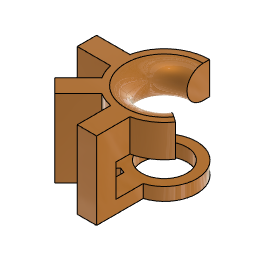
Exercise-18 v0 (Autodesk Fusion 360 design; units mm, degrees)
Autodesk Fusion 360 part; units mm, degrees
sketch "Sketch1" plane through (0, 0, 0) normal (1, 0, 0) x (0, 1, 0)
  line L0 (0, -2.5) -> (1, -2.5)
  line L1 (1, -2.5) -> (1, 2.5)
  line L2 (1, 2.5) -> (0, 2.5)
  arc A0 (0, 2.5) -> (0, -2.5) centre (0, 0) ccw
  line L3 (-6, 5) -> (-6, -5)
  dimension "d1" = 5
  dimension "d2" = 1
  dimension "d3" = 5
  dimension "d4" = 6
  constraint coincident A0.centre origin
  constraint horizontal L0
  constraint vertical L1
  constraint horizontal L2
  constraint vertical L3
  measures "d1" diameter of A0
  measures "d2" distance of L0.start L0.end
  measures "d3" distance of L0.start L2.end
  measures "d4" distance of A0.centre L3
revolve "Revolve1" add sketch "Sketch1" angle 235 about axis through (0, -6, 5) along (0, 0, 1) makes body 1
sketch "Sketch2" plane through (0, 0, 2.5) normal (0, 0, 1) x (-1, 0, 0)
  line L0 (0, 0) -> (0, -1)
  arc A0 (0, -1) -> (-5.7341, 10.015) centre (0, 6) ccw
  line L1 (-5.7341, 10.015) -> (-4.9149, 9.4415)
  arc A1 (0, 0) -> (-4.9149, 9.4415) centre (0, 6) ccw
  line L2 (6, 7.5) -> (12, 7.5)
  line L3 (12, 7.5) -> (12, 4.5)
  line L4 (12, 4.5) -> (6, 4.5)
  line L5 (6, 4.5) -> (6, 7.5)
  line L6 (12, 7.5) -> (9, 7.5)
  line L7 (9, 7.5) -> (9, 4.5)
  line L8 (9, 4.5) -> (12, 4.5)
  line L9 (12, 4.5) -> (12, 7.5)
  line L10 (7.4246, 15.5459) -> (5.3033, 13.4246)
  line L11 (5.3033, 13.4246) -> (7.4246, 11.3033)
  line L12 (9.5459, 13.4246) -> (7.4246, 15.5459)
  line L13 (7.4246, 11.3033) -> (9.5459, 13.4246)
  line L14 (7.4246, 15.5459) -> (9.5459, 13.4246)
  line L15 (5.3033, 9.182) -> (3.182, 11.3033)
  line L16 (3.182, 11.3033) -> (7.4246, 15.5459)
  line L17 (9.5459, 13.4246) -> (5.3033, 9.182)
  line L18 (-1.5, 18) -> (-1.5, 15)
  line L19 (-1.5, 15) -> (1.5, 15)
  line L20 (1.5, 18) -> (-1.5, 18)
  line L21 (1.5, 15) -> (1.5, 18)
  line L22 (-1.5, 18) -> (1.5, 18)
  line L23 (1.5, 12) -> (-1.5, 12)
  line L24 (-1.5, 12) -> (-1.5, 18)
  line L25 (1.5, 18) -> (1.5, 12)
  dimension "d6" = 6
  dimension "d7" = 3
  dimension "d8" = 12
  dimension "d9" = 1.5
  dimension "d10" = 3
  dimension "d11" = 3
  dimension "d13" = 90
  constraint horizontal L2
  constraint vertical L3
  constraint horizontal L4
  constraint vertical L5
  constraint horizontal L6
  constraint vertical L7
  constraint horizontal L8
  constraint vertical L9
  measures "d6" distance of L2.start L2.end
  measures "d7" distance of L2.start L4.end
  measures "d8" distance of A0.centre L3
  measures "d9" distance of A0.centre L4
  measures "d10" distance of L2.end L6.end
  measures "d11" distance of L2.end L3.end
extrude "Extrude1" add sketch "Sketch2" against normal blind 12 separate body contours L2 L3 L4 L6 L7 L8 L9 | L10 L11 L12 L13 L14 L16 L17 | L18 L19 L20 L21 L22 L24 L25 makes body 2 at (-6.0104, -14.1317, -5.5) makes body 3 at (0.5, -15, -1.5) makes body 4 at (-9, -6.5, -1.5)
extrude "Extrude2" add sketch "Sketch2" against normal blind 5 contours A0 L2 L4 L7 | A0 L11 L16 L17 | A0 L19 L24 L25 bodies 1 2 3 4
sketch "Sketch3" plane through (0, 0, -9.5) normal (0, 0, -1) x (1, 0, 0)
  line L0 (-1.5, 15) -> (1.5, 15)
  line L1 (1.5, 15) -> (1.5, 18)
  line L2 (1.5, 18) -> (-1.5, 18)
  line L3 (-1.5, 18) -> (-1.5, 15)
  line L4 (-12, 7.5) -> (-6.8374, 7.5)
  line L5 (-6.8374, 4.5) -> (-12, 4.5)
  line L6 (-12, 4.5) -> (-12, 7.5)
  arc A0 (-6.8374, 4.5) -> (0, -1) centre (0, 6) ccw
  line L7 (-1.5, 18) -> (-1.5, 12.8374)
  line L8 (1.5, 18) -> (-1.5, 18)
  line L9 (1.5, 12.8374) -> (1.5, 18)
  arc A1 (-1.5, 12.8374) -> (-3.7741, 11.8954) centre (0, 6) ccw
  line L10 (-9.5459, 13.4246) -> (-5.8954, 9.7741)
  line L11 (-7.4246, 15.5459) -> (-9.5459, 13.4246)
  line L12 (-3.7741, 11.8954) -> (-7.4246, 15.5459)
  arc A2 (-5.8954, 9.7741) -> (-6.8374, 7.5) centre (0, 6) ccw
  arc A3 (5.7341, 10.015) -> (1.5, 12.8374) centre (0, 6) ccw
  line L13 (0, -1) -> (0, 0)
  line L14 (4.9149, 9.4415) -> (5.7341, 10.015)
  line L15 (0, 0) -> (0, 2.5)
  line L16 (2.867, 8.0075) -> (4.9149, 9.4415)
  arc A4 (2.867, 8.0075) -> (0, 2.5) centre (0, 6) ccw
  circle A5 centre (0, 6) radius 3.5
  circle A6 centre (0, 6) radius 5
  line L17 (1.5, 12.8374) -> (-1.5, 12.8374)
  line L18 (-1.5, 12.8374) -> (-1.5, 9.8374)
  line L19 (-1.5, 9.8374) -> (1.5, 9.8374)
  line L20 (1.5, 9.8374) -> (1.5, 12.8374)
  line L21 (-3.7741, 7.6528) -> (-1.6528, 9.7741)
  line L22 (-1.6528, 9.7741) -> (-3.7741, 11.8954)
  line L23 (-5.8954, 9.7741) -> (-3.7741, 7.6528)
  line L24 (-3.7741, 11.8954) -> (-5.8954, 9.7741)
  line L25 (-3.8374, 4.5) -> (-3.8374, 7.5)
  line L26 (-3.8374, 7.5) -> (-6.8374, 7.5)
  line L27 (-6.8374, 4.5) -> (-3.8374, 4.5)
  line L28 (-6.8374, 7.5) -> (-6.8374, 4.5)
  dimension "d18" = 7
  dimension "d19" = 10
  dimension "d20" = 3
  dimension "d21" = 3
  dimension "d23" = 90
  constraint concentric A0 A5
  constraint concentric A0 A6
  constraint horizontal L17
  constraint vertical L18
  constraint horizontal L19
  constraint vertical L20
  constraint coincident L9.start A3.end
  measures "d18" diameter of A5
  measures "d19" diameter of A6
  measures "d20" distance of L9.start L7.end
  measures "d21" distance of L9.start L19.end
extrude "Extrude3" add sketch "Sketch3" against normal blind 2 contours L0 L7 L9 L17 | A6 L17 L18 L20 | L10 L11 L12 L24 | A6 L22 L23 L24 | L15 L16 A4 A5 A6 L18 L19 L20 L21 L22 L23 L25 L26 L27 | A6 L18 L19 L20 | A6 L21 L22 L23 | L15 L16 A5 A6 | L4 L5 L6 L28 | A6 L26 L27 L28 | A6 L25 L26 L27 bodies 1
